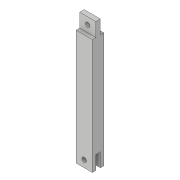
# Autodesk Inventor part: LD_holder_p4
Saved by Autodesk Inventor 2019 (Build 230136000, 136)
## iProperties
Created: 2020-08-30
Part Number: LD_holder_p4
Material: Generic
Document SubType Name: Modeling
Designer: LIU
Density: 1 g/cm^3
Appearance: Default
Author: LIU
Autodesk Inventor part; units mm, degrees
ref_plane "YZ Plane" through (0, 0, 0) normal (1, 0, 0) x (0, 1, 0)
ref_plane "XZ Plane" through (0, 0, 0) normal (0, 1, 0) x (-1, 0, 0)
ref_plane "XY Plane" through (0, 0, 0) normal (0, 0, 1) x (1, 0, 0)
sketch "Sketch1" plane through (0, 0, 0) normal (0, 1, 0) x (-1, 0, 0)
  line L0 (-3.5, 2.5) -> (3.5, 2.5)
  line L1 (3.5, 2.5) -> (3.5, -2.5)
  line L2 (3.5, -2.5) -> (-3.5, -2.5)
  line L3 (-3.5, -2.5) -> (-3.5, 2.5)
  line L4 (-3.5, 2.5) -> (3.5, -2.5) construction
  line L5 (3.5, 2.5) -> (-3.5, -2.5) construction
  point P0 (0, 0)
  dimension "d0" = 5
  dimension "d1" = 7
  constraints: 12 end point, 2 midpoint, 2 parallel, 1 horizontal, 1 perpendicular
  measures "d0" distance of L0.end L1.end
  measures "d1" distance of L1.end L2.end
extrude "Extrusion1" add sketch "Sketch1" along normal blind 50
sketch "Sketch2" plane through (0, 50, 0) normal (0, 1, 0) x (1, 0, 0)
  line L0 (-3.5, -2.5) -> (3.5, -2.5) projected
  line L1 (3.5, -2.5) -> (3.5, 2.5) projected
  line L2 (3.5, 2.5) -> (-3.5, 2.5) projected
  line L3 (-3.5, -2.5) -> (3.5, -2.5)
  line L4 (3.5, -2.5) -> (3.5, -0.98)
  line L5 (3.5, -0.98) -> (-3.5, -0.98)
  line L6 (-3.5, -0.98) -> (-3.5, -2.5)
  line L7 (-3.5, 2.5) -> (3.5, 2.5)
  line L8 (3.5, 2.5) -> (3.5, 0.98)
  line L9 (3.5, 0.98) -> (-3.5, 0.98)
  line L10 (-3.5, 0.98) -> (-3.5, 2.5)
  point P0 (0, 0)
  dimension "d4" = 1.52
  dimension "d5" = 1.52
  constraints: 16 end point, 4 parallel, 2 horizontal, 2 perpendicular, 2 point on line
  measures "d4" distance between parallel lines of L0 L5
  measures "d5" distance between parallel lines of L2 L9
extrude "Extrusion2" cut sketch "Sketch2" against normal blind 6
sketch "Sketch3" plane through (-3.5, 50, 0.98) normal (0, 0, 1) x (1, 0, 0)
  line L0 (0, 0) -> (7, 0) projected
  line L1 (7, 0) -> (7, -6) projected
  circle A0 centre (3.5, -3) radius 1
  point P0 (3.5, -50)
  dimension "d8" = 2
  dimension "d9" = 3.5
  dimension "d10" = 3
  constraints: 1 centre point
  measures "d8" diameter of A0
  measures "d9" distance from line of L1 A0.centre
  measures "d10" distance from line of L0 A0.centre
extrude "Extrusion3" cut sketch "Sketch3" against normal through all
sketch "Sketch4" plane through (0, 0, 0) normal (0, -1, 0) x (1, 0, 0)
  line L0 (3.5, 2.5) -> (-3.5, 2.5) projected
  line L1 (-3.5, 2.5) -> (-3.5, -2.5) projected
  line L2 (-3.5, -2.5) -> (3.5, -2.5) projected
  line L3 (3.5, 0.98) -> (3.5, -0.98) projected
  line L4 (-3.5, 2.5) -> (3.5, 2.5)
  line L5 (3.5, 2.5) -> (3.5, 1.02)
  line L6 (3.5, 1.02) -> (-3.5, 1.02)
  line L7 (-3.5, 1.02) -> (-3.5, 2.5)
  line L8 (-3.5, -2.5) -> (3.5, -2.5) projected
  line L9 (3.5, -2.5) -> (-3.5, -2.5)
  line L10 (-3.5, -2.5) -> (-3.5, -1.02)
  line L11 (-3.5, -1.02) -> (3.5, -1.02)
  line L12 (3.5, -1.02) -> (3.5, -2.5)
  point P0 (0, 0)
  dimension "d13" = 1.48
  dimension "d14" = 1.48
  constraints: 16 end point, 4 parallel, 2 horizontal, 2 perpendicular, 2 point on line
  measures "d13" distance between parallel lines of L0 L6
  measures "d14" distance between parallel lines of L2 L11
extrude "Extrusion4" add sketch "Sketch4" along normal blind 6
sketch "Sketch5" plane through (-3.5, 0, 1.02) normal (0, 0, -1) x (1, 0, 0)
  line L0 (7, 0) -> (0, 0) projected
  line L1 (7, 0) -> (7, 6) projected
  circle A0 centre (3.5, 3) radius 1
  point P0 (3.5, 0)
  dimension "d17" = 3
  dimension "d18" = 3.5
  dimension "d19" = 2
  constraints: 1 centre point
  measures "d17" distance from line of L0 A0.centre
  measures "d18" distance from line of A0.centre L1
  measures "d19" diameter of A0
extrude "Extrusion6" cut sketch "Sketch5" along normal through all both and the other way through all
body "Solid1"
